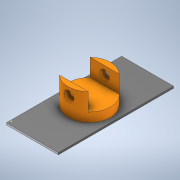
# Autodesk Inventor part: Part1
Saved by Autodesk Inventor 2021 (Build 250183000, 183)
## iProperties
Created: 2021-07-24
Part Number: Part1
Material: Generic
Document SubType Name: Modeling
Designer: aksha
Density: 1 g/cm^3
Appearance: Default
Author: aksha
Autodesk Inventor part; units mm, degrees
ref_plane "YZ Plane" through (0, 0, 0) normal (1, 0, 0) x (0, 1, 0)
ref_plane "XZ Plane" through (0, 0, 0) normal (0, 1, 0) x (-1, 0, 0)
ref_plane "XY Plane" through (0, 0, 0) normal (0, 0, 1) x (1, 0, 0)
sketch "Sketch1" plane through (0, 0, 0) normal (0, 1, 0) x (-1, 0, 0)
  line L0 (6.793, 18.7845) -> (-263.207, 18.7845)
  line L1 (-263.207, 18.7845) -> (-263.207, -581.2155)
  line L2 (-263.207, -581.2155) -> (6.793, -581.2155)
  line L3 (6.793, -581.2155) -> (6.793, 18.7845)
  point P0 (0, 0)
  dimension "d0" = 270
  dimension "d1" = 600
  constraints: 8 end point, 2 parallel, 1 horizontal, 1 perpendicular
  measures "d0" distance of L2.end L1.end
  measures "d1" distance of L1.end L0.end
extrude "Extrusion1" add sketch "Sketch1" along normal blind 10
sketch "Sketch2" plane through (0, 10, 0) normal (0, 1, 0) x (1, 0, 0)
  point P0 (0, 0)
sketch "Sketch3" plane through (0, 10, 0) normal (0, 1, 0) x (1, 0, 0)
  circle A0 centre (131.029, 274.6873) radius 110
  point P0 (0, 0)
  dimension "d4" = 220
  constraints: 1 centre point
  measures "d4" diameter of A0
extrude "Extrusion2" add sketch "Sketch3" along normal blind 140
sketch "Sketch4" plane through (131.029, 150, -274.6873) normal (0, 1, 0) x (1, 0, 0)
  circle A0 centre (0, 0) radius 110 projected
  line L0 (-75.1726, -80.3062) -> (75.1726, -80.3062)
  line L1 (75.1726, -80.3062) -> (75.1726, 80.3062)
  line L2 (75.1726, 80.3062) -> (-75.1726, 80.3062)
  line L3 (-75.1726, 80.3062) -> (-75.1726, -80.3062)
  line L4 (-75.1726, -80.3062) -> (75.1726, 80.3062) construction
  line L5 (75.1726, -80.3062) -> (-75.1726, 80.3062) construction
  arc A1 (-75.1726, 80.3062) -> (-75.1726, -80.3062) centre (0, 0) ccw
  arc A2 (75.1726, -80.3062) -> (75.1726, 80.3062) centre (0, 0) ccw
  point P0 (-131.029, -274.6873)
  point P1 (-75.1726, 80.3062)
  point P2 (75.1726, -80.3062)
  constraints: 12 end point, 5 point on circle, 2 centre point, 2 concentric, 2 midpoint, 2 parallel, 1 horizontal, 1 perpendicular
extrude "Extrusion3" cut sketch "Sketch4" against normal blind 92 contours A0 L1 | L1 L0 L3 L2 | L3 A0
sketch "Sketch5" plane through (206.2016, 150, -194.3811) normal (0, 0, -1) x (-1, 0, 0)
  circle A0 centre (72.7519, -41.0963) radius 25
  point P0 (206.2016, -150)
  dimension "d9" = 50
  constraints: 1 centre point
  measures "d9" diameter of A0
extrude "Extrusion4" cut sketch "Sketch5" against normal blind 92
sketch "Sketch6" plane through (55.8564, 150, -354.9935) normal (0, 0, 1) x (1, 0, 0)
  circle A0 centre (74.775, -43.4815) radius 25
  point P0 (-55.8564, -150)
  dimension "d12" = 50
  constraints: 1 centre point
  measures "d12" diameter of A0
extrude "Extrusion5" cut sketch "Sketch6" against normal blind 92
body "Solid1"
